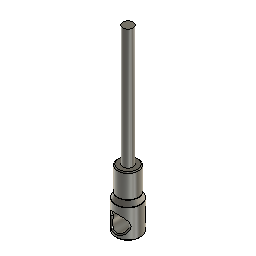
Connie (Autodesk Fusion 360 archive; units mm, degrees)
design "Fastening screw 1"
Autodesk Fusion 360 part; units mm, degrees
sketch "Sketch1" plane through (0, 0, 0) normal (0, 1, 0) x (1, 0, 0)
  line L0 (0, 0) -> (-6, 0)
  line L1 (-6, 0) -> (-6, -14)
  line L2 (0, 0) -> (0, -28)
  line L3 (-2.5, -28) -> (-5, -28)
  line L4 (-5, -28) -> (-5, -16.5)
  line L5 (-6, -14) -> (-5, -16.5)
  line L6 (0, -28) -> (0, -86)
  line L7 (0, -86) -> (-2.5, -86)
  line L8 (-2.5, -86) -> (-2.5, -28)
  dimension "d1" = 6
  dimension "d2" = 14
  dimension "d3" = 28
  dimension "d4" = 5
  dimension "d6" = 58
  dimension "d7" = 2.5
  constraint coincident L0.start L2.start
  constraint horizontal L0
  constraint perpendicular L0 L1
  constraint perpendicular L0 L2
  constraint perpendicular L2 L3
  constraint perpendicular L3 L4
  constraint perpendicular L3 L6
  constraint perpendicular L6 L7
  measures "d1" distance of L0.start L0.end
  measures "d2" distance of L0.end L1.end
  measures "d3" distance of L0.start L2.end
  measures "d4" distance of L2.end L3.end
  measures "d6" distance of L2.end L6.end
  measures "d7" distance of L6.end L7.end
revolve "Revolve1" add sketch "Sketch1" angle 360 about axis through (0, 0, 0) along (0, 0, 1)
ref_plane "WorkPlane1" through (0, 6, 0) normal (0, 1, 0) x (0, 0, 1)
sketch "Sketch3" plane through (0, 6, 0) normal (0, 1, 0) x (1, 0, 0)
  line L0 (6, 0) -> (-6, 0)
  line L1 (0, 0) -> (0, -2)
  line L2 (0, -2) -> (0, -6)
  circle A0 centre (0, -6) radius 4
  dimension "d10" = 2
  dimension "d11" = 4
  constraint coincident L1.start origin
  constraint perpendicular L0 L1
  constraint parallel L1 L2
  constraint coincident L2.end A0.centre
  constraint coincident L1.end A0
  measures "d10" distance of L1.start L1.end
  measures "d11" distance of L1.end L2.end
extrude "Extrude1" cut sketch "Sketch3" against normal blind 57
fillet "Fillet1" radius 0.5 3 faces at (-4.9938, 0.2492, 20.3333) (-2.8333, -4.9075, 14.8333) (-5.9702, 0.5974, 4.6667)

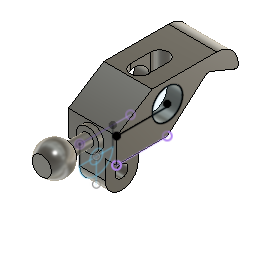
design "Fixed Arm"
Autodesk Fusion 360 part; units mm, degrees
sketch "Sketch1" plane through (0, 0, 0) normal (1, 0, 0) x (0, 1, 0)
  line L0 (0, 0) -> (0, 10)
  line L1 (0, 0) -> (20, 0)
  line L2 (20, 0) -> (36, 0)
  line L3 (0, 10) -> (14, 10)
  line L4 (14, 10) -> (14, 19)
  line L5 (0, 10) -> (14, 19)
  line L6 (48, 19) -> (14, 19)
  line L7 (36, 0) -> (36, 14)
  line L8 (36, 14) -> (20, 0)
  line L9 (48, 14) -> (48, 19)
  line L10 (48, 14) -> (48, 9)
  line L11 (48, 9) -> (36, 14)
  dimension "d1" = 10
  dimension "d2" = 20
  dimension "d3" = 16
  dimension "d5" = 14
  dimension "d6" = 9
  dimension "d15" = 5
  constraint coincident L0.start L1.start
  constraint vertical L0
  constraint perpendicular L0 L1
  constraint parallel L1 L2
  constraint perpendicular L0 L3
  constraint perpendicular L3 L4
  constraint perpendicular L4 L6
  constraint perpendicular L6 L9
  measures "d1" distance of L0.start L0.end
  measures "d2" distance of L0.start L1.end
  measures "d3" distance of L1.end L2.end
  measures "d5" distance of L0.end L3.end
  measures "d6" distance of L3.end L4.end
  measures "d15" distance of L9.start L10.end
extrude "Extrude1" add sketch "Sketch1" along normal blind 19 contours L0 L1 L3 L4 L6 L8 L9 L10 L11 | L3 L4 L5
fillet "Fillet3" radius 1 1 edges at (9.5, 48, 9)
fillet "Fillet4" radius 8.5 1 edges at (9.5, 48, 19)
fillet "Fillet5" radius 2 1 edges at (9.5, 36, 14)
sketch "Sketch2" plane through (19, 0, 0) normal (1, 0, 0) x (0, 1, 0)
  line L0 (0, 0) -> (20, 0)
  line L1 (0, 10) -> (20, 10)
  line L2 (20, 10) -> (20, 11)
  circle A0 centre (20, 11) radius 6
  point P0 (0, 10)
  dimension "d22" = 20
  dimension "d26" = 1
  dimension "d27" = 12
  constraint coincident P0 L1.start
  constraint parallel L0 L1
  constraint perpendicular L1 L2
  constraint coincident L2.end A0.centre
  measures "d22" distance of P0 L1.end
  measures "d26" distance of L1.end L2.end
  measures "d27" diameter of A0
extrude "Extrude3" cut sketch "Sketch2" against normal blind 44
sketch "Sketch3" plane through (0, 0, 19) normal (0, 0, 1) x (-1, 0, 0)
ref_plane "WorkPlane1" through (4.5, 0, 0) normal (1, 0, 0) x (0, 1, 0)
sketch "Sketch4" plane through (4.5, 0, 0) normal (1, 0, 0) x (0, 1, 0)
  line L0 (0, 0) -> (20, 0)
  line L1 (0, 0) -> (0, -7.5)
  line L2 (13, -7.5) -> (13, 0)
  line L3 (0, 0) -> (13, 0)
  line L4 (6.5, -7.5) -> (6.5, -17)
  line L5 (0, -7.5) -> (13, -7.5)
  arc A0 (0, -7.5) -> (13, -7.5) centre (6.5, -7.5) ccw
  circle A1 centre (6.5, -7.5) radius 2.5
  dimension "d33" = 6.5
  dimension "d37" = 5
  constraint coincident L0.start L1.start
  constraint perpendicular L0 L1
  constraint coincident L0 L2.end
  constraint perpendicular L0 L2
  constraint tangent L2 A0
  constraint perpendicular L2 L5
  constraint concentric A0 A1
  measures "d33" radius of A0
  measures "d37" diameter of A1
extrude "Extrude4" add sketch "Sketch4" along normal blind 10
extrude "Extrude5" cut sketch "Sketch4" along normal blind 17 contours L5 A1 | L4 L5 A1 | L4 L5 A1
sketch "Sketch5" plane through (0, 0, 19) normal (0, 0, 1) x (-1, 0, 0)
  line L0 (0, -14) -> (-19, -14)
  line L1 (0, -39.5) -> (-19, -39.5)
  line L2 (-9.5, -14) -> (-9.5, -39.5)
  line L3 (-9.5, -14) -> (-9.5, -15)
  line L4 (0, -20) -> (-19, -20)
  line L5 (-9.5, -15) -> (-9.5, -18.5)
  line L6 (-13, -18.5) -> (-13, -26.5)
  arc A0 (-13, -26.5) -> (-6, -26.5) centre (-9.5, -26.5) ccw
  line L7 (-6, -26.5) -> (-6, -18.5)
  arc A1 (-6, -18.5) -> (-13, -18.5) centre (-9.5, -18.5) ccw
  line L8 (-9.5, -18.5) -> (-9.5, -26.5) construction
  dimension "d40" = 1
  dimension "d41" = 3.5
  dimension "d42" = 7
  dimension "d43" = 8
  constraint midpoint L0 L2.start
  constraint midpoint L1 L2.end
  constraint perpendicular L0 L3
  constraint perpendicular L4 L5
  constraint tangent L6 A0
  constraint tangent A0 L7
  constraint parallel L6 L7
  constraint tangent L7 A1
  constraint tangent L6 A1
  constraint perpendicular L4 L8
  constraint coincident L5.end A1.centre
  measures "d40" distance of L2.start L3.end
  measures "d41" distance of L3.end L5.end
  measures "d42" diameter of A0
  measures "d43" distance of L5.end A0.centre
extrude "Extrude6" cut sketch "Sketch5" against normal blind 30
ref_plane "WorkPlane2" through (9.5, 0, 0) normal (1, 0, 0) x (0, 1, 0)
sketch "Sketch7" plane through (9.5, 0, 0) normal (1, 0, 0) x (0, 1, 0)
  line L0 (0, 0) -> (0, 10)
  line L1 (0, 5) -> (-2, 5)
  line L2 (-2, 7.5) -> (-2, 9.5)
  line L3 (-2, 9.5) -> (0, 9.5)
  line L4 (0, 5) -> (0, 9.5)
  line L5 (-2, 5) -> (-10, 5)
  line L6 (-10, 5) -> (-10, 7.5)
  line L7 (-9.2718, 7.5) -> (-2, 7.5)
  line L8 (-10, 5) -> (-20, 5)
  line L9 (-10, 7.5) -> (-10, 8.75)
  line L10 (-20, 5) -> (-20, 8.75)
  arc A0 (-10, 8.75) -> (-20, 8.75) centre (-15, 5) ccw
  line L11 (-9.2718, 7.5) -> (-10, 7.5)
  dimension "d47" = 2
  dimension "d48" = 4.5
  dimension "d49" = 8
  dimension "d50" = 2.5
  dimension "d51" = 10
  dimension "d52" = 12.5
  constraint midpoint L0 L1.start
  constraint perpendicular L0 L1
  constraint perpendicular L1 L2
  constraint coincident L0 L3.end
  constraint perpendicular L0 L3
  constraint perpendicular L2 L5
  constraint perpendicular L5 L6
  constraint perpendicular L2 L7
  constraint perpendicular L6 L8
  constraint midpoint L8 A0.centre
  constraint perpendicular L7 L9
  constraint perpendicular L8 L10
  constraint perpendicular L9 L11
  measures "d47" distance of L1.start L1.end
  measures "d48" distance of L1.end L2.end
  measures "d49" distance of L1.end L5.end
  measures "d50" distance of L5.end L6.end
  measures "d51" distance of L5.end L8.end
  measures "d52" diameter of A0
revolve "Revolve1" add sketch "Sketch7" angle 360 about axis through (9.5, -10, 5) along (0, -1, 0)

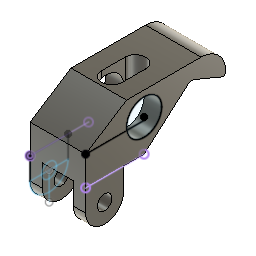
design "Free Arm"
Autodesk Fusion 360 part; units mm, degrees
sketch "Sketch1" plane through (0, 0, 0) normal (1, 0, 0) x (0, 1, 0)
  line L0 (0, 0) -> (0, 10)
  line L1 (0, 0) -> (20, 0)
  line L2 (20, 0) -> (36, 0)
  line L3 (0, 10) -> (14, 10)
  line L4 (14, 10) -> (14, 19)
  line L5 (0, 10) -> (14, 19)
  line L6 (48, 19) -> (14, 19)
  line L7 (36, 0) -> (36, 14)
  line L8 (36, 14) -> (20, 0)
  line L9 (48, 14) -> (48, 19)
  line L10 (48, 14) -> (48, 9)
  line L11 (48, 9) -> (36, 14)
  dimension "d1" = 10
  dimension "d2" = 20
  dimension "d3" = 16
  dimension "d5" = 14
  dimension "d6" = 9
  dimension "d15" = 5
  constraint coincident L0.start L1.start
  constraint vertical L0
  constraint perpendicular L0 L1
  constraint parallel L1 L2
  constraint perpendicular L0 L3
  constraint perpendicular L3 L4
  constraint perpendicular L4 L6
  constraint perpendicular L6 L9
  measures "d1" distance of L0.start L0.end
  measures "d2" distance of L0.start L1.end
  measures "d3" distance of L1.end L2.end
  measures "d5" distance of L0.end L3.end
  measures "d6" distance of L3.end L4.end
  measures "d15" distance of L9.start L10.end
extrude "Extrude1" add sketch "Sketch1" along normal blind 19 contours L0 L1 L3 L4 L6 L8 L9 L10 L11 | L3 L4 L5
fillet "Fillet3" radius 1 1 edges at (9.5, 48, 9)
fillet "Fillet4" radius 8.5 1 edges at (9.5, 48, 19)
fillet "Fillet5" radius 2 1 edges at (9.5, 36, 14)
sketch "Sketch2" plane through (19, 0, 0) normal (1, 0, 0) x (0, 1, 0)
  line L0 (0, 0) -> (20, 0)
  line L1 (0, 10) -> (20, 10)
  line L2 (20, 10) -> (20, 11)
  circle A0 centre (20, 11) radius 6
  point P0 (0, 10)
  dimension "d22" = 20
  dimension "d26" = 1
  dimension "d27" = 12
  constraint coincident P0 L1.start
  constraint parallel L0 L1
  constraint perpendicular L1 L2
  constraint coincident L2.end A0.centre
  measures "d22" distance of P0 L1.end
  measures "d26" distance of L1.end L2.end
  measures "d27" diameter of A0
extrude "Extrude3" cut sketch "Sketch2" against normal blind 44
sketch "Sketch3" plane through (0, 0, 19) normal (0, 0, 1) x (-1, 0, 0)
ref_plane "WorkPlane1" through (0, 0, 0) normal (1, 0, 0) x (0, 1, 0)
sketch "Sketch4" plane through (0, 0, 0) normal (1, 0, 0) x (0, 1, 0)
  line L0 (0, 0) -> (20, 0)
  line L1 (0, 0) -> (0, -7.5)
  line L2 (13, -7.5) -> (13, 0)
  line L3 (0, 0) -> (13, 0)
  line L4 (6.5, -7.5) -> (6.5, -17)
  line L5 (0, -7.5) -> (13, -7.5)
  arc A0 (0, -7.5) -> (13, -7.5) centre (6.5, -7.5) ccw
  circle A1 centre (6.5, -7.5) radius 2.5
  dimension "d33" = 6.5
  dimension "d37" = 5
  constraint coincident L0.start L1.start
  constraint perpendicular L0 L1
  constraint coincident L0 L2.end
  constraint perpendicular L0 L2
  constraint tangent L2 A0
  constraint perpendicular L2 L5
  constraint concentric A0 A1
  constraint coincident L0.start L1
  measures "d33" radius of A0
  measures "d37" diameter of A1
sketch "Sketch5" plane through (0, 0, 19) normal (0, 0, 1) x (-1, 0, 0)
  line L0 (0, -14) -> (-19, -14)
  line L1 (0, -39.5) -> (-19, -39.5)
  line L2 (-9.5, -14) -> (-9.5, -39.5)
  line L3 (-9.5, -14) -> (-9.5, -15)
  line L4 (0, -20) -> (-19, -20)
  line L5 (-9.5, -15) -> (-9.5, -18.5)
  line L6 (-13, -18.5) -> (-13, -26.5)
  arc A0 (-13, -26.5) -> (-6, -26.5) centre (-9.5, -26.5) ccw
  line L7 (-6, -26.5) -> (-6, -18.5)
  arc A1 (-6, -18.5) -> (-13, -18.5) centre (-9.5, -18.5) ccw
  line L8 (-9.5, -18.5) -> (-9.5, -26.5) construction
  dimension "d40" = 1
  dimension "d41" = 3.5
  dimension "d42" = 7
  dimension "d43" = 8
  constraint midpoint L0 L2.start
  constraint midpoint L1 L2.end
  constraint perpendicular L0 L3
  constraint perpendicular L4 L5
  constraint tangent L6 A0
  constraint tangent A0 L7
  constraint parallel L6 L7
  constraint tangent L7 A1
  constraint tangent L6 A1
  constraint perpendicular L4 L8
  constraint coincident L5.end A1.centre
  measures "d40" distance of L2.start L3.end
  measures "d41" distance of L3.end L5.end
  measures "d42" diameter of A0
  measures "d43" distance of L5.end A0.centre
extrude "Extrude6" cut sketch "Sketch5" against normal blind 30
extrude "Extrude7" add sketch "Sketch4" along normal blind 4.2 contours L0 L1 L2 L3 L5 A1 | L4 L5 A0 A1 | L4 L5 A0 A1
ref_plane "WorkPlane3" through (9.5, 0, 0) normal (1, 0, 0) x (0, 1, 0)
sketch "Sketch8" plane through (19, 0, 0) normal (1, 0, 0) x (0, 1, 0)
  arc A0 (0, -7.5) -> (13, -7.5) centre (6.5, -7.5) ccw
  line L0 (0, 0) -> (0, -7.5)
  line L1 (13, 0) -> (13, -7.5)
  line L2 (0, 0) -> (13, 0)
  arc A1 (0, -7.5) -> (13, -7.5) centre (6.5, -7.5) ccw
  point P0 (13, 0)
  point P1 (13, 0)
  constraint coincident L0.start L2.start
  constraint coincident A0.start L0.end
  constraint coincident P1 P0
  constraint coincident A0.end L1.end
  constraint concentric A0 A1
extrude "Extrude8" add sketch "Sketch8" against normal blind 4.2
sketch "Sketch9" plane through (14.8, 0, 0) normal (-1, 0, 0) x (0, -1, 0)
  circle A0 centre (-6.5, -7.5) radius 2.5
  point P0 (-6.5, -7.5)
  constraint coincident P0 A0.centre
extrude "Extrude9" cut sketch "Sketch9" against normal blind 16

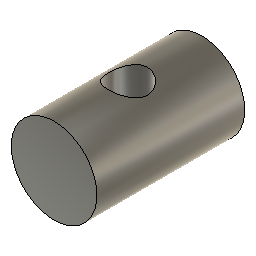
design "Spacer pins"
Autodesk Fusion 360 part; units mm, degrees
sketch "Sketch1" plane through (0, 0, 0) normal (0, 1, 0) x (1, 0, 0)
  circle A0 centre (0, 0) radius 5.5
  dimension "d1" = 11
  constraint coincident A0.centre origin
  measures "d1" diameter of A0
extrude "Extrude1" add sketch "Sketch1" along normal blind 19
ref_plane "WorkPlane1" through (0, 0, 5.5) normal (0, 0, 1) x (1, 0, 0)
sketch "Sketch2" plane through (0, 0, 5.5) normal (0, 0, 1) x (1, 0, 0)
  line L0 (5.5, 19) -> (-5.5, 19)
  line L1 (0, 0) -> (0, 9.5)
  circle A0 centre (0, 9.5) radius 2.5
  dimension "d5" = 9.5
  dimension "d6" = 5
  constraint coincident L1.start origin
  constraint perpendicular L0 L1
  constraint coincident L1.end A0.centre
  measures "d5" distance of L1.start L1.end
  measures "d6" diameter of A0
extrude "Extrude2" cut sketch "Sketch2" against normal blind 19

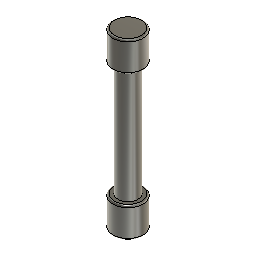
design "Fastening screw 2"
Autodesk Fusion 360 part; units mm, degrees
sketch "Sketch1" plane through (0, 0, 0) normal (1, 0, 0) x (0, 1, 0)
  line L0 (0, 0) -> (0, 52)
  line L1 (0, 0) -> (-4.5, 0)
  line L2 (-4.5, 0) -> (-4.5, 9)
  line L3 (-4.5, 9) -> (-3, 9)
  line L4 (-3, 9) -> (-3, 43)
  line L5 (-3, 52) -> (0, 52)
  line L6 (0, 52) -> (-4.5, 52)
  line L7 (-4.5, 52) -> (-4.5, 43)
  line L8 (-4.5, 43) -> (-3, 43)
  dimension "d1" = 52
  dimension "d2" = 4.5
  dimension "d3" = 9
  dimension "d5" = 4.5
  dimension "d6" = 9
  constraint coincident L0.start L1.start
  constraint vertical L0
  constraint perpendicular L0 L1
  constraint perpendicular L1 L2
  constraint perpendicular L2 L3
  constraint perpendicular L0 L5
  constraint perpendicular L0 L6
  constraint perpendicular L6 L7
  constraint perpendicular L4 L8
  measures "d1" distance of L0.start L0.end
  measures "d2" distance of L0.start L1.end
  measures "d3" distance of L1.end L2.end
  measures "d5" distance of L0.end L6.end
  measures "d6" distance of L6.end L7.end
revolve "Revolve1" add sketch "Sketch1" angle 360 about axis through (0, 0, 0) along (0, 0, 1)
fillet "Fillet1" radius 0.5 2 faces at (-0.2243, -4.4944, 49) (-0.2243, -4.4944, 3)
